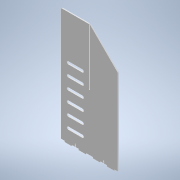
# Autodesk Inventor part: Korpus
Saved by Autodesk Inventor 2021.1 (Build 251245010, 245A)
## iProperties
Created: 2023-03-13
Part Number: Korpus
Material: Типовые
Document SubType Name: Modeling
Designer: User
Density: 1 g/cm^3
Appearance: По умолчанию
Author: User
Autodesk Inventor part; units mm, degrees
ref_plane "YZ Plane" through (0, 0, 0) normal (1, 0, 0) x (0, 1, 0)
ref_plane "XZ Plane" through (0, 0, 0) normal (0, 1, 0) x (-1, 0, 0)
ref_plane "XY Plane" through (0, 0, 0) normal (0, 0, 1) x (1, 0, 0)
sketch "Эскиз1" plane through (0, 0, 0) normal (0, 0, 1) x (1, 0, 0)
  line L0 (0, 0) -> (0, 595)
  line L1 (5, 600) -> (147, 600)
  line L2 (153, 600) -> (298.5355, 454.4645)
  line L3 (300, 450.9289) -> (300, 0)
  line L4 (300, 0) -> (281.25, 0)
  line L5 (281.25, 0) -> (281.25, -6)
  line L6 (281.25, -6) -> (243.75, -6)
  line L7 (243.75, -6) -> (243.75, 0)
  line L8 (243.75, 0) -> (206.25, 0)
  line L9 (206.25, 0) -> (206.25, -6)
  line L10 (206.25, -6) -> (168.75, -6)
  line L11 (168.75, -6) -> (168.75, 0)
  line L12 (168.75, 0) -> (131.25, 0)
  line L13 (131.25, 0) -> (131.25, -6)
  line L14 (131.25, -6) -> (93.75, -6)
  line L15 (93.75, -6) -> (93.75, 0)
  line L16 (93.75, 0) -> (56.25, 0)
  line L17 (56.25, 0) -> (56.25, -6)
  line L18 (56.25, -6) -> (18.75, -6)
  line L19 (18.75, -6) -> (18.75, 0)
  line L20 (18.75, 0) -> (0, 0)
  line L21 (18.75, 0) -> (-18.75, 0) construction
  line L22 (281.25, 0) -> (318.75, 0) construction
  line L23 (153, 600) -> (147, 600) construction
  line L24 (150, 600) -> (150, 0) construction
  line L25 (0, 300) -> (150, 300) construction
  line L26 (150, 300) -> (300, 300) construction
  arc A0 (37.5, 375) -> (37.5, 360) centre (37.5, 367.5) ccw
  line L27 (37.5, 360) -> (112.5, 360)
  line L28 (37.5, 375) -> (112.5, 375)
  line L29 (75, 375) -> (75, 360) construction
  arc A1 (112.5, 360) -> (112.5, 375) centre (112.5, 367.5) ccw
  line L30 (37.5, 367.5) -> (0, 367.5) construction
  line L31 (112.5, 367.5) -> (150, 367.5) construction
  line L32 (37.5, 300) -> (112.5, 300)
  arc A2 (112.5, 300) -> (112.5, 315) centre (112.5, 307.5) ccw
  line L33 (37.5, 315) -> (112.5, 315)
  arc A3 (37.5, 315) -> (37.5, 300) centre (37.5, 307.5) ccw
  line L34 (37.5, 240) -> (112.5, 240)
  arc A4 (112.5, 240) -> (112.5, 255) centre (112.5, 247.5) ccw
  line L35 (37.5, 255) -> (112.5, 255)
  arc A5 (37.5, 255) -> (37.5, 240) centre (37.5, 247.5) ccw
  line L36 (37.5, 180) -> (112.5, 180)
  arc A6 (112.5, 180) -> (112.5, 195) centre (112.5, 187.5) ccw
  line L37 (37.5, 195) -> (112.5, 195)
  arc A7 (37.5, 195) -> (37.5, 180) centre (37.5, 187.5) ccw
  line L38 (37.5, 120) -> (112.5, 120)
  arc A8 (112.5, 120) -> (112.5, 135) centre (112.5, 127.5) ccw
  line L39 (37.5, 135) -> (112.5, 135)
  arc A9 (37.5, 135) -> (37.5, 120) centre (37.5, 127.5) ccw
  line L40 (37.5, 60) -> (112.5, 60)
  arc A10 (112.5, 60) -> (112.5, 75) centre (112.5, 67.5) ccw
  line L41 (37.5, 75) -> (112.5, 75)
  arc A11 (37.5, 75) -> (37.5, 60) centre (37.5, 67.5) ccw
  line L42 (153, 300) -> (147, 300)
  line L43 (153, 300) -> (153, 600)
  line L44 (147, 300) -> (147, 600)
  arc A12 (300, 450.9289) -> (298.5355, 454.4645) centre (295, 450.9289) ccw
  arc A13 (5, 600) -> (0, 595) centre (5, 595) ccw
  point P0 (0, 600)
  point P1 (300, 453)
  point P2 (75, 300)
  point P3 (75, 315)
  point P4 (75, 240)
  point P5 (75, 255)
  point P6 (75, 180)
  point P7 (75, 195)
  point P8 (75, 120)
  point P9 (75, 135)
  point P10 (75, 60)
  point P11 (75, 75)
  dimension "d0" = 6
  dimension "d1" = 300
  dimension "d3" = 135
  dimension "d4" = 153
  dimension "d7" = 15
  dimension "d8" = 75
  dimension "d9" = 225
  dimension "d12" = 60
  dimension "d17" = 6
  dimension "d18" = 5
  dimension "d19" = 5
  dimension "d20" = 600
  constraints: 91 end point, 28 point on circle, 18 point on line, 14 centre point, 12 equal length, 12 perpendicular, 9 midpoint, 7 horizontal, 5 tangent, 4 vertical, 3 horizontal alignment, 3 vertical alignment, 1 parallel, 1 symmetric about line, 61 other
  measures "d0" distance of L4.end L5.end
  measures "d1" distance between parallel lines of L3 L0
  measures "d3" angle of L1 L2
  measures "d4" distance of point (0, 600) L2.start
  measures "d7" distance between parallel lines of L27 L28
  measures "d8" distance of L27.start L27.end
  measures "d9" distance between parallel lines of L1 L28
  measures "d12" distance of L27.start L32.start
  measures "d17" distance of L42.start L42.end
  measures "d18" radius of A12
  measures "d19" radius of A13
  measures "d20" distance between parallel lines of L20 L1
extrude "Корпус" add sketch "Эскиз1" along normal blind 6
sketch "Эскиз2" plane through (0, 0, 0) normal (0, 0, -1) x (-1, 0, 0)
  line L0 (-227, -6) -> (-227, 0) construction
  line L1 (-223, -6) -> (-223, 0) construction
  line L2 (-227, 0) -> (-227, 5.95)
  line L3 (-227, 5.95) -> (-228.4, 5.95)
  line L4 (-228.4, 5.95) -> (-228.4, 9.05)
  line L5 (-228.4, 9.05) -> (-227, 9.05)
  line L6 (-227, 9.05) -> (-227, 15)
  line L7 (-227, 15) -> (-223, 15)
  line L8 (-223, 15) -> (-223, 9.05)
  line L9 (-223, 9.05) -> (-221.6, 9.05)
  line L10 (-221.6, 9.05) -> (-221.6, 5.95)
  line L11 (-221.6, 5.95) -> (-223, 5.95)
  line L12 (-223, 5.95) -> (-223, 0)
  line L13 (-153, 55) -> (-153, 595) construction
  line L14 (-147, 55) -> (-147, 595) construction
  line L15 (-153, 595) -> (-147, 595) construction
  line L16 (-153, 55) -> (-147, 55) construction
  line L17 (-150, 595) -> (-150, 55) construction
  line L18 (-227, 0) -> (-223, 0)
  line L19 (-73, 0) -> (-73, 5.95)
  line L20 (-73, 5.95) -> (-71.6, 5.95)
  line L21 (-71.6, 5.95) -> (-71.6, 9.05)
  line L22 (-71.6, 9.05) -> (-73, 9.05)
  line L23 (-73, 9.05) -> (-73, 15)
  line L24 (-73, 15) -> (-77, 15)
  line L25 (-77, 15) -> (-77, 9.05)
  line L26 (-77, 9.05) -> (-78.4, 9.05)
  line L27 (-78.4, 9.05) -> (-78.4, 5.95)
  line L28 (-78.4, 5.95) -> (-77, 5.95)
  line L29 (-77, 5.95) -> (-77, 0)
  line L30 (-73, 0) -> (-77, 0)
  point P0 (0, 0)
  dimension "d21" = 15
  dimension "d22" = 3.1
  dimension "d23" = 6.8
  constraints: 58 end point, 14 point on line, 12 symmetric about line, 7 perpendicular, 3 vertical, 2 collinear, 2 midpoint, 1 horizontal, 1 parallel, 4 other
  measures "d21" distance from line of L7 L1.end
  measures "d22" distance between parallel lines of L11 L9
  measures "d23" distance between parallel lines of L10 L4
extrude "Пазы" cut sketch "Эскиз2" against normal blind 6
equation "\"d4\" = 0.5 * d0 + 0.5 * d1"
equation "\"d8\" = 0.25 * d1"
equation "\"d9\" = 15 * d7"
equation "\"d12\" = 4 * d7"
equation "\"d17\" = d0"
equation "\"d5\" = d0"
equation "\"d24\" = d0"
